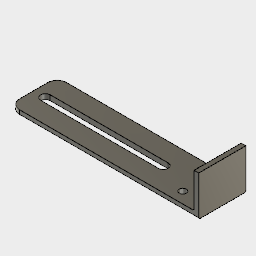
CableChain-10x10-Y-Carriage v1 (Autodesk Fusion 360 design; units mm, degrees)
Autodesk Fusion 360 part; units mm, degrees
sketch "Sketch1" plane through (0, 0, 0) normal (0, 0, 1) x (1, 0, 0)
  line L0 (0, 0) -> (80, 0)
  line L1 (80, 0) -> (80, 20)
  line L2 (80, 20) -> (0, 20)
  line L3 (0, 20) -> (0, 0)
  line L4 (80, 20) -> (60, 20)
  line L5 (60, 20) -> (60, 0)
  line L6 (60, 0) -> (80, 0)
  line L7 (80, 0) -> (80, 20)
  line L8 (80, 20) -> (78, 20)
  line L9 (78, 20) -> (78, 0)
  line L10 (78, 0) -> (80, 0)
  line L11 (80, 0) -> (80, 20)
  line L12 (55, 12) -> (5, 12)
  arc A0 (5, 12) -> (5, 8) centre (5, 10) ccw
  line L13 (5, 8) -> (55, 8)
  arc A1 (55, 8) -> (55, 12) centre (55, 10) ccw
  line L14 (55, 10) -> (5, 10) construction
  point P0 (30, 10)
  dimension "d1" = 80
  dimension "d2" = 20
  dimension "d3" = 20
  dimension "d4" = 2
  dimension "d6" = 4
  measures "d1" distance of L0.start L0.end
  measures "d2" distance of L0.start L2.end
  measures "d3" distance of L1.end L0.end
  measures "d4" distance of L1.end L8.end
  measures "d6" diameter of A0
extrude "Extrude1" add sketch "Sketch1" along normal blind 2.2 contours L0 L2 L3 L5 | L0 L2 L4 L5 L6 L9
extrude "Extrude2" add sketch "Sketch1" along normal blind 15 contours L0 L1 L2 L4 L6 L7 L8 L9 L10 L11
chamfer "Chamfer1" distance 0.5 angle 45 1 edges at (78, 10, 2.2)
fillet "Fillet1" radius 4 2 edges at (0, 0, 1.1) (0, 20, 1.1)
fillet "Fillet2" radius 0.5 5 edges at (42, 20, 0) (1.1716, 18.8284, 0) (0, 10, 0) (1.1716, 1.1716, 0) (42, 0, 0)
sketch "Sketch2" plane through (0, 0, 2.2) normal (0, 0, 1) x (-1, 0, 0)
  arc A0 (-4, -20) -> (0, -16) centre (-4, -16) ccw
  line L0 (0, -16) -> (0, -4)
  arc A1 (0, -4) -> (-4, 0) centre (-4, -4) ccw
  line L1 (-4, 0) -> (-77.5, 0)
  line L2 (-77.5, 0) -> (-77.5, -20)
  line L3 (-77.5, -20) -> (-4, -20)
  arc A2 (-55, -8) -> (-55, -12) centre (-55, -10) ccw
  line L4 (-55, -8) -> (-5, -8)
  arc A3 (-5, -12) -> (-5, -8) centre (-5, -10) ccw
  line L5 (-5, -12) -> (-55, -12)
  line L6 (-77.5, 0) -> (-59.5, 0)
  line L7 (-59.5, 0) -> (-59.5, -20)
  line L8 (-59.5, -20) -> (-77.5, -20)
  line L9 (-77.5, -20) -> (-77.5, 0)
  circle A4 centre (-68.5, -4.7) radius 1.5
  circle A5 centre (-68.5, -12.7) radius 1.5
  dimension "d14" = 18
  dimension "d15" = 3
  dimension "d16" = 9
  dimension "d17" = 20
  dimension "d18" = 4.7
  dimension "d19" = 3
  dimension "d20" = 8
  measures "d14" distance of L1.end L6.end
  measures "d15" diameter of A4
  measures "d16" distance of L7 A4.centre
  measures "d17" distance of L1.end L2.end
  measures "d18" distance of L6 A4.centre
  measures "d19" diameter of A5
  measures "d20" distance of A4.centre A5.centre
extrude "Extrude3" cut sketch "Sketch2" against normal blind 10 contours A4 | A5
extrude "Extrude4" add 1 faces at (78.6667, 13.3333, 15) along direction (0, 0, 1) blind 2
